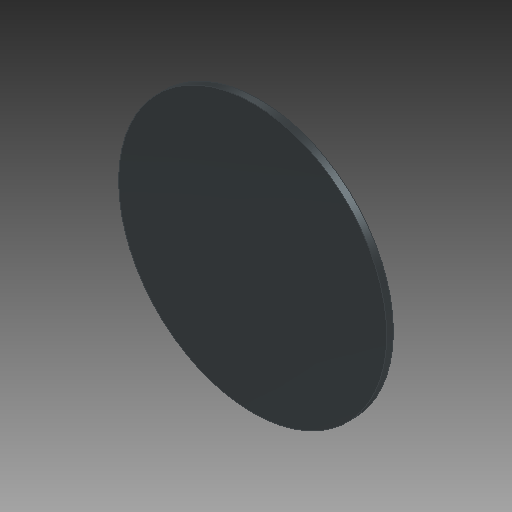
# Autodesk Inventor part: lid
Saved by Autodesk Inventor 2020 (Build 240168000, 168)
## iProperties
Created: 2024-12-06
Part Number: lid
Material: Полиэтилен, низкая плотность
Document SubType Name: Modeling
Designer: Ivan
Density: 0.894 g/cm^3
Appearance: Чугун серый
Author: Ivan
Autodesk Inventor part; units mm, degrees
ref_plane "YZ Plane" through (0, 0, 0) normal (1, 0, 0) x (0, 1, 0)
ref_plane "XZ Plane" through (0, 0, 0) normal (0, 1, 0) x (-1, 0, 0)
ref_plane "XY Plane" through (0, 0, 0) normal (0, 0, 1) x (1, 0, 0)
derived "mirror2.ipt"
sketch "Эскиз2" plane through (0, 0, 0) normal (0, 0, -1) x (-1, 0, 0)
  circle A0 centre (0, 0) radius 57.8311
  point P0 (0, 0)
sketch "Эскиз3" plane through (0, 0, 0) normal (0, 0, 1) x (1, 0, 0)
  circle A0 centre (0, 0) radius 57.8311 construction
  circle A1 centre (0, 0) radius 58.1311
  circle A2 centre (0, 0) radius 80
  point P0 (0, 0)
  dimension "d1" = 115.6622
  dimension "d2" = 116.2622
  dimension "d3" = 160
  constraints: 2 centre point, 2 coincident
  measures "d1" diameter of A0
  measures "d2" diameter of A1
  measures "d3" diameter of A2
extrude "Выдавливание1" add sketch "Эскиз3" along normal blind 4 contours A1 | A2
extrude "Выдавливание2" cut sketch "Эскиз3" along normal blind 1 contours A1
sketch "Эскиз5" plane through (0, 0, 0) normal (0, 0, -1) x (-1, 0, 0)
  circle A0 centre (0, 0) radius 60
  circle A1 centre (0, 0) radius 65
  dimension "d8" = 120
  dimension "d9" = 130
  constraints: 2 centre point, 2 coincident
  measures "d8" diameter of A0
  measures "d9" diameter of A1
extrude "Выдавливание3" cut sketch "Эскиз5" against normal blind 2
